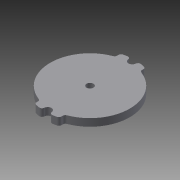
# Autodesk Inventor part: Front Outer Endcap
Saved by Autodesk Inventor 2013 SP1 (Build 170176100, 176)
## iProperties
Created: 2013-05-24
Part Number: Front Outer Endcap
Material: Generic
Document SubType Name: Modeling
Designer: Eric
Density: 1 g/cm^3
Author: Eric
Autodesk Inventor part; units mm, degrees
ref_plane "YZ Plane" through (0, 0, 0) normal (1, 0, 0) x (0, 1, 0)
ref_plane "XZ Plane" through (0, 0, 0) normal (0, 1, 0) x (-1, 0, 0)
ref_plane "XY Plane" through (0, 0, 0) normal (0, 0, 1) x (1, 0, 0)
sketch "Sketch1" plane through (0, 0, 0) normal (0, 0, 1) x (1, 0, 0)
  circle A0 centre (0, 0) radius 1.4
  line L0 (5, 16.5227) -> (5, 15.906)
  line L1 (5, -15.906) -> (5, -16.5227)
  line L2 (-5, -16.5227) -> (-5, -15.906)
  line L3 (-5, 15.906) -> (-5, 16.5227)
  arc A1 (-5.6471, 14.9703) -> (-5.6471, -14.9703) centre (0, 0) ccw
  arc A2 (5.6471, -14.9703) -> (5.6471, 14.9703) centre (0, 0) ccw
  arc A3 (-5.6471, 14.9703) -> (-5, 15.906) centre (-6, 15.906) ccw
  arc A4 (-4.2353, 17.4946) -> (-5, 16.5227) centre (-4, 16.5227) ccw
  arc A5 (5, 16.5227) -> (4.2353, 17.4946) centre (4, 16.5227) ccw
  arc A6 (5, 15.906) -> (5.6471, 14.9703) centre (6, 15.906) ccw
  arc A7 (5.6471, -14.9703) -> (5, -15.906) centre (6, -15.906) ccw
  arc A8 (4.2353, -17.4946) -> (5, -16.5227) centre (4, -16.5227) ccw
  arc A9 (-5, -16.5227) -> (-4.2353, -17.4946) centre (-4, -16.5227) ccw
  arc A10 (-5, -15.906) -> (-5.6471, -14.9703) centre (-6, -15.906) ccw
  arc A11 (-1.4959, 16.8897) -> (1.4959, 16.8897) centre (0, 17) ccw
  arc A12 (1.4959, -16.8897) -> (-1.4959, -16.8897) centre (0, -17) ccw
  arc A13 (-4.2353, -17.4946) -> (-2.6399, -17.8054) centre (0, 0) ccw
  arc A14 (2.6399, -17.8054) -> (4.2353, -17.4946) centre (0, 0) ccw
  arc A15 (4.2353, 17.4946) -> (2.6399, 17.8054) centre (0, 0) ccw
  arc A16 (-2.6399, 17.8054) -> (-4.2353, 17.4946) centre (0, 0) ccw
  arc A17 (-1.4959, 16.8897) -> (-2.6399, 17.8054) centre (-2.4932, 16.8162) ccw
  arc A18 (2.6399, 17.8054) -> (1.4959, 16.8897) centre (2.4932, 16.8162) ccw
  arc A19 (-2.6399, -17.8054) -> (-1.4959, -16.8897) centre (-2.4932, -16.8162) ccw
  arc A20 (1.4959, -16.8897) -> (2.6399, -17.8054) centre (2.4932, -16.8162) ccw
  point P0 (5, -17.2916)
  point P1 (-5, -17.2916)
  point P2 (5, 15.1987)
  point P3 (5, -15.1987)
  point P4 (-5, -15.1987)
  point P5 (-5, 15.1987)
  point P6 (-5, 17.2916)
  point P7 (5, 17.2916)
  dimension "d3" = 2.8
  dimension "d9" = 1
  dimension "d12" = 16
  dimension "d13" = 16
  dimension "d14" = 10
  dimension "d15" = 10
  dimension "d16" = 5
  dimension "d17" = 5
  dimension "d18" = 3
  dimension "d19" = 17
  dimension "d20" = 3
  dimension "d21" = 17
  dimension "d22" = 1
  constraints: 44 point on circle, 21 centre point, 20 tangent, 10 equal radius, 8 end point, 8 point on line, 4 parallel, 3 coincident
  measures "d3" diameter of A0
  measures "d9" radius of A3
  measures "d12" radius of A1
  measures "d13" radius of A2
  measures "d14" distance between parallel lines of L0 L3
  measures "d15" distance between parallel lines of L1 L2
  measures "d16" distance from line of A0.centre L0
  measures "d17" distance from line of A0.centre L2
  measures "d18" diameter of A11
  measures "d19" distance of A1.centre A11.centre
  measures "d20" diameter of A12
  measures "d21" distance of A12.centre point (0, 0)
  measures "d22" radius of A17
extrude "Extrusion1" add sketch "Sketch1" along normal blind 3
body "Solid1"
